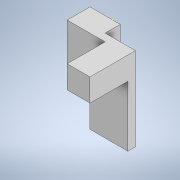
# Autodesk Inventor part: Součást1
Saved by Autodesk Inventor 2022 (Build 260153000, 153)
## iProperties
Created: 2022-03-14
Part Number: Součást1
Material: Všeobecné
Document SubType Name: Modeling
Designer: Šimon
Density: 1 g/cm^3
Appearance: Výchozí
Author: Šimon
Autodesk Inventor part; units mm, degrees
ref_plane "YZ Plane" through (0, 0, 0) normal (1, 0, 0) x (0, 1, 0)
ref_plane "XZ Plane" through (0, 0, 0) normal (0, 1, 0) x (-1, 0, 0)
ref_plane "XY Plane" through (0, 0, 0) normal (0, 0, 1) x (1, 0, 0)
sketch "Náčrt3" plane through (0, 0, 0) normal (0, 0, 1) x (1, 0, 0)
  line L0 (0, 0) -> (25, 0)
  line L1 (25, 0) -> (25, 55)
  line L2 (25, 55) -> (-15, 55)
  line L3 (-15, 55) -> (-15, 15)
  line L4 (-15, 15) -> (0, 15)
  line L5 (0, 15) -> (0, 0)
  dimension "d7" = 25
  dimension "d8" = 55
  dimension "d9" = 40
  dimension "d10" = 40
  dimension "d11" = 15
  constraints: 12 end point, 3 perpendicular, 2 horizontal
  measures "d7" distance of L0.start L0.end
  measures "d8" distance of L0.end L1.end
  measures "d9" distance of L1.end L2.end
  measures "d10" distance of L2.end L3.end
  measures "d11" distance of L3.end L4.end
extrude "Vysunutí2" add sketch "Náčrt3" along normal blind 15
sketch "Náčrt4" plane through (0, 0, 15) normal (0, 0, 1) x (1, 0, 0)
  line L0 (25, 55) -> (-15, 55) projected
  line L1 (25, 55) -> (10, 55)
  line L2 (10, 55) -> (10, 40)
  line L3 (10, 40) -> (25, 40)
  line L4 (25, 40) -> (25, 55)
  point P0 (0, 0)
  dimension "d14" = 15
  dimension "d15" = 15
  constraints: 8 end point, 2 parallel, 1 horizontal, 1 perpendicular
  measures "d14" distance of L3.end L2.end
  measures "d15" distance of L2.end L1.end
extrude "Vysunutí3" add sketch "Náčrt4" along normal blind 25
sketch "Náčrt5" plane through (-15, 55, 0) normal (0, 1, 0) x (1, 0, 0)
  point P0 (15, 0)
sketch "Náčrt6" plane through (-15, 55, 0) normal (0, 1, 0) x (1, 0, 0)
  line L0 (40, 0) -> (0, 0) projected
  line L1 (40, 0) -> (20, 0)
  line L2 (20, 0) -> (20, -10)
  line L3 (20, -10) -> (40, -10)
  line L4 (40, -10) -> (40, 0)
  point P0 (15, 0)
  dimension "d18" = 20
  dimension "d19" = 10
  constraints: 8 end point, 2 parallel, 1 horizontal, 1 perpendicular
  measures "d18" distance of L3.end L2.end
  measures "d19" distance of L2.end L1.end
extrude "Vysunutí4" cut sketch "Náčrt6" against normal through all
